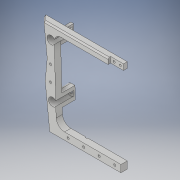
# Autodesk Inventor part: iPadGolf6Holder
Saved by Autodesk Inventor 2017 (Build 210142000, 142)
## iProperties
Created: 2022-11-09
Part Number: iPadGolf6Holder
Material: Generic
Document SubType Name: Modeling
Designer: khonsu
Density: 1 g/cm^3
Appearance: Default
Author: khonsu
Autodesk Inventor part; units mm, degrees
ref_plane "YZ Plane" through (0, 0, 0) normal (1, 0, 0) x (0, 1, 0)
ref_plane "XZ Plane" through (0, 0, 0) normal (0, 1, 0) x (-1, 0, 0)
sketch "Sketch1" plane through (0, 0, 0) normal (0, 0, 1) x (1, 0, 0)
  circle A0 centre (0, 0) radius 2.9
  line L0 (0, 0) -> (-2.42, 85.0556) construction
  line L1 (0, 0) -> (85.09, 0) construction
  line L2 (0, 0) -> (0, 165.0391) construction
  line L3 (-2.42, 85.0556) -> (0, 85.0556) construction
  circle A1 centre (-2.42, 85.0556) radius 2.9
  line L4 (0.48, 85.0556) -> (112.48, 85.0556) construction
  line L5 (112.48, 85.0556) -> (114.98, 85.0556) construction
  line L6 (-1.82, 94.7556) -> (2.68, 94.7556)
  line L7 (2.68, 85.6556) -> (2.68, 75.3556)
  line L8 (2.68, 75.3556) -> (-8.82, 75.3556)
  line L9 (-8.82, 75.3556) -> (-8.82, 87.7556)
  line L10 (-8.82, 87.6845) -> (1.18, 87.6845) construction
  line L11 (-1.4, -9.9) -> (5.7, -9.9)
  line L12 (5.7, -9.9) -> (5.7, 9.9)
  line L13 (5.7, 9.9) -> (-1.4, 9.9)
  line L14 (-6.4, 4.9) -> (-6.4, -4.9)
  arc A2 (-1.4, 9.9) -> (-6.4, 4.9) centre (-1.4, 4.9) ccw
  arc A3 (-6.4, -4.9) -> (-1.4, -9.9) centre (-1.4, -4.9) ccw
  line L15 (-1.82, 94.7556) -> (-8.82, 87.7556)
  line L16 (13.68, 96.6556) -> (114.98, 96.6556)
  line L17 (19.7, -32.2) -> (114.98, -32.2)
  line L18 (85.98, 105.8556) -> (114.98, 105.8556)
  line L19 (110.98, -43.7444) -> (114.98, -43.7444)
  line L20 (110.98, -43.7444) -> (-4.52, -43.7444)
  line L21 (110.98, -43.7444) -> (226.48, -43.7444) construction
  line L22 (85.98, 105.8556) -> (-20.72, 105.8556)
  line L23 (85.98, 105.8556) -> (192.68, 105.8556) construction
  line L24 (-20.72, 105.8556) -> (-4.52, -43.7444)
  line L25 (2.68, 96.6556) -> (2.68, 94.7556)
  line L26 (5.7, -18.2) -> (5.7, -9.9)
  arc A4 (13.68, 96.6556) -> (2.68, 85.6556) centre (13.68, 85.6556) ccw
  arc A5 (5.7, -18.2) -> (19.7, -32.2) centre (19.7, -18.2) ccw
  line L27 (114.98, 105.8556) -> (114.98, -43.7444)
  line L28 (2.68, 85.6556) -> (2.68, 94.7556)
  point P0 (-8.82, 94.7556)
  point P1 (5.7, -32.2)
  point P2 (-8.82, -58.1944)
  dimension "d5" = 5.8
  dimension "d0" = 5.8
  dimension "d1" = 85.09
  dimension "d3" = 2.42
  dimension "d4" = 0
  dimension "d6" = 112
  dimension "d7" = 2.5
  dimension "d10" = 9.7
  dimension "d11" = 6.4
  dimension "d12" = 5.1
  dimension "d13" = 9.7
  dimension "d16" = 0
  dimension "d18" = 6.4
  dimension "d19" = 9.9
  dimension "d20" = 9.9
  dimension "d21" = 5.7
  dimension "d22" = 5
  dimension "d23" = 7
  dimension "d24" = 7
  dimension "d25" = 1.9
  dimension "d26" = 0
  dimension "d27" = 0
  dimension "d28" = 22.3
  dimension "d29" = 0
  dimension "d30" = 0
  dimension "d31" = 149.6
  dimension "d32" = 9.2
  dimension "d33" = 4
  dimension "d34" = 0
  dimension "d35" = 115.5
  dimension "d36" = 180
  dimension "d37" = 29
  dimension "d38" = 0
  dimension "d39" = 106.7
  dimension "d40" = 180
  dimension "d41" = 11
  dimension "d42" = 14
  constraints: 58 end point, 13 horizontal, 9 tangent, 8 point on circle, 7 point on line, 5 centre point, 4 parallel, 4 perpendicular, 3 equal length, 2 coincident, 1 equal radius, 1 horizontal alignment, 1 vertical, 2 other
  measures "d0" diameter of A0
  measures "d1" distance of L0.start L0.end
  measures "d3" distance of L0.end L3.end
  measures "d4" distance from line of L2 L3.end
  measures "d6" distance of L4.start L4.end
  measures "d7" distance of L4.end L5.end
  measures "d10" distance from line of L6 point (-2.42, 85.056)
  measures "d11" distance from line of L9 point (-2.42, 85.056)
  measures "d12" distance from line of point (-2.42, 85.056) L7
  measures "d13" distance from line of L8 point (-2.42, 85.056)
  measures "d16" distance from line of L9 L10.start
  measures "d18" distance from line of L0.start L14
  measures "d19" distance from line of L11 L0.start
  measures "d20" distance from line of L13 L0.start
  measures "d21" distance from line of L12 L0.start
  measures "d22" radius of A2
  measures "d23" distance of L6.start point (-8.82, 94.756)
  measures "d24" distance of L9.end point (-8.82, 94.756)
  measures "d25" distance between parallel lines of L6 L16
  measures "d26" distance from line of L7 L25.start
  measures "d27" horizontal distance of L16.end L5.end
  measures "d28" distance between parallel lines of L11 L17
  measures "d29" distance from line of L12 point (5.7, -32.2)
  measures "d30" horizontal distance of L5.end L17.end
  measures "d31" distance between parallel lines of L19 L18
  measures "d32" distance between parallel lines of L16 L18
  measures "d33" distance of L19.start L19.end
  measures "d34" horizontal distance of L17.end L19.end
  measures "d35" distance of L19.start L20.end
  measures "d36" angle of L20 L21
  measures "d37" distance of L18.start L18.end
  measures "d38" horizontal distance of L16.end L18.end
  measures "d39" distance of L18.start L22.end
  measures "d40" angle of L22 L23
  measures "d41" radius of A4
  measures "d42" radius of A5
sketch "Sketch2" plane through (0, 0, 0) normal (1, 0, 0) x (0, 1, 0)
  line L0 (90.8641, 0) -> (90.8641, 21.12) construction
  line L1 (0, 0) -> (0, 31.12) construction
  dimension "d8" = 21.12
  dimension "d9" = 31.12
  constraints: 4 end point, 2 vertical
  measures "d8" distance of L0.start L0.end
  measures "d9" distance of L1.start L1.end
ref_plane "Work Plane2" through (0, 0, 31.12) normal (0, 0, 1) x (1, 0, 0)
sketch "Sketch4" plane through (0, 0, 31.12) normal (0, 0, 1) x (1, 0, 0)
  line L0 (3.18, 120.306) -> (114.98, 120.306)
  line L1 (114.98, 120.306) -> (114.98, -58.194)
  line L2 (114.98, -58.194) -> (3.18, -58.194)
  line L3 (-8.82, -46.194) -> (-8.82, 108.306)
  arc A0 (3.18, 120.306) -> (-8.82, 108.306) centre (3.18, 108.306) ccw
  arc A1 (-8.82, -46.194) -> (3.18, -58.194) centre (3.18, -46.194) ccw
  point P0 (0, 0)
  point P1 (-8.82, 120.306)
  dimension "d53" = 123.8
  dimension "d54" = 178.5
  dimension "d55" = 12
  dimension "d56" = 120.306
  dimension "d57" = 114.98
  constraints: 8 end point, 4 point on circle, 4 tangent, 2 centre point, 2 parallel, 2 point on line, 1 equal radius, 1 horizontal, 1 perpendicular
  measures "d53" distance of point (-8.82, 120.306) L0.end
  measures "d54" distance of L0.end L1.end
  measures "d55" radius of A0
  measures "d56" distance from line of point (0, 0) L0
  measures "d57" distance from line of L1 point (0, 0)
extrude "Extrusion1" add sketch "Sketch4" along normal blind 6.2
sketch "Sketch5" plane through (0, 0, 37.32) normal (0, 0, 1) x (1, 0, 0)
  line L0 (-30.2901, 140.4978) -> (261.1035, 140.4978) construction
  line L1 (261.1035, 140.4978) -> (261.1035, -78.1737) construction
  line L2 (261.1035, -78.1737) -> (-30.2901, -78.1737) construction
  line L3 (-30.2901, -78.1737) -> (-30.2901, 140.4978) construction
  line L4 (2.9472, 95.7116) -> (21.4756, 95.7116)
  line L5 (21.4756, 95.7116) -> (21.4756, 55.8918)
  line L6 (21.4756, 55.8918) -> (2.9472, 55.8918)
  line L7 (2.9472, 55.8918) -> (2.9472, 95.7116)
  line L8 (-5.1793, 84.9846) -> (1.4844, 84.9846)
  line L9 (1.4844, 84.9846) -> (1.4844, 67.7564)
  line L10 (1.4844, 67.7564) -> (-5.1793, 67.7564)
  line L11 (-5.1793, 67.7564) -> (-5.1793, 84.9846)
  line L12 (-5.1793, -10.2579) -> (1.4844, -10.2579)
  line L13 (1.4844, -10.2579) -> (1.4844, -27.486)
  line L14 (1.4844, -27.486) -> (-5.1793, -27.486)
  line L15 (-5.1793, -27.486) -> (-5.1793, -10.2579)
  line L16 (5.5477, 19.16) -> (22.6133, 19.16)
  line L17 (22.6133, 19.16) -> (22.6133, -33.4996)
  line L18 (22.6133, -33.4996) -> (5.5477, -33.4996)
  line L19 (5.5477, -33.4996) -> (5.5477, 19.16)
  line L20 (8.6767, 118.5205) -> (34.3813, 118.5205)
  line L21 (34.3813, 118.5205) -> (34.3813, 113.4913)
  line L22 (34.3813, 113.4913) -> (8.6767, 113.4913)
  line L23 (8.6767, 113.4913) -> (8.6767, 118.5205)
  line L24 (-1.8474, 113.4913) -> (21.4756, 113.4913)
  line L25 (21.4756, 113.4913) -> (21.4756, 89.4631)
  line L26 (21.4756, 89.4631) -> (-1.8474, 89.4631)
  line L27 (-1.8474, 89.4631) -> (-1.8474, 113.4913)
  arc A0 (3.4892, 119.7039) -> (-8.3493, 107.663) centre (3.3651, 107.9857) ccw
  line L28 (-8.82, 108.306) -> (-8.82, -46.194) projected
  line L29 (3.18, -58.194) -> (114.98, -58.194) projected
  arc A1 (-8.82, -46.194) -> (3.18, -58.194) centre (3.7792, -45.5948) ccw
  line L30 (-8.82, -46.194) -> (-8.82, 108.306)
  line L31 (114.98, 120.306) -> (3.18, 120.306) projected
  line L32 (3.18, 120.306) -> (85.0606, 120.306)
  line L33 (3.18, -58.194) -> (79.7167, -58.194)
  point P0 (0, 0)
  constraints: 54 end point, 13 equal length, 6 horizontal, 6 perpendicular, 6 point on line, 4 point on circle, 2 centre point, 2 other
extrude "Extrusion2" add sketch "Sketch1" along normal blind 2 contours L6 L28 L7 L8 L9 L15 | A3 L14 A2 L13 L12 L11
sketch "Sketch6" plane through (0, 0, 2) normal (0, 0, 1) x (1, 0, 0)
  circle A0 centre (-2.42, 85.0556) radius 2.9 projected
  circle A1 centre (-2.42, 85.0556) radius 6
  line L0 (-8.82, 87.7556) -> (-8.82, 75.3556) projected
  line L1 (-8.82, 75.3556) -> (2.68, 75.3556) projected
  line L2 (2.68, 81.5556) -> (2.68, 75.3556)
  line L3 (2.68, 75.3556) -> (-8.82, 75.3556)
  line L4 (-8.82, 75.3556) -> (-8.82, 81.5556)
  line L5 (2.68, 94.7556) -> (-1.82, 94.7556) projected
  line L6 (2.68, 94.7556) -> (-1.82, 94.7556)
  line L7 (-1.82, 94.7556) -> (-5.32, 91.2556)
  line L8 (-1.82, 94.7556) -> (-8.82, 87.7556) projected
  line L9 (-5.32, 91.2556) -> (2.68, 91.2556)
  line L10 (2.68, 75.3556) -> (2.68, 94.7556) projected
  line L11 (2.68, 94.7556) -> (2.68, 91.2556)
  circle A2 centre (0, 0) radius 2.9 projected
  arc A3 (5.7, 1.8735) -> (5.7, -1.8735) centre (0, 0) ccw
  arc A4 (-1.4, 9.9) -> (-6.4, 4.9) centre (-1.4, 4.9) ccw projected
  arc A5 (-1.4, 9.9) -> (-6.4, 4.9) centre (-1.4, 4.9) ccw
  arc A6 (-6.4, -4.9) -> (-1.4, -9.9) centre (-1.4, -4.9) ccw projected
  arc A7 (-6.4, -4.9) -> (-1.4, -9.9) centre (-1.4, -4.9) ccw
  line L12 (5.7, 9.9) -> (-1.4, 9.9) projected
  line L13 (5.7, 9.9) -> (-1.4, 9.9)
  line L14 (-6.4, 4.9) -> (-6.4, -4.9)
  line L15 (-1.4, -9.9) -> (5.7, -9.9)
  line L16 (5.7, -9.9) -> (5.7, 9.9)
  line L17 (-8.82, 81.5556) -> (-7.2934, 81.5556)
  line L18 (2.4534, 81.5556) -> (2.68, 81.5556)
  line L19 (-6.4, 4.9) -> (-6.4, -4.9) projected
  line L20 (-6.4, 4.9) -> (-6.4, -4.9)
  line L21 (-1.4, -9.9) -> (5.7, -9.9) projected
  line L22 (-1.4, -9.9) -> (5.7, -9.9)
  dimension "d103" = 12
  dimension "d104" = 12
  constraints: 30 end point, 12 point on circle, 6 parallel, 4 centre point, 4 perpendicular, 3 collinear, 3 horizontal, 3 point on line, 2 coincident, 2 concentric, 2 midpoint
  measures "d103" diameter of A1
  measures "d104" diameter of A3
extrude "Extrusion3" add sketch "Sketch6" along normal blind 19 contours A1 L18 L2 L1 L0 L17 | L9 L7 L5 L10 | A3 L16 L15 A6 L14 A4 L12
sketch "Sketch7" plane through (0, 0, 21) normal (0, 0, 1) x (1, 0, 0)
  line L0 (114.98, 105.8556) -> (-20.72, 105.8556)
  line L1 (-20.72, 105.8556) -> (-4.52, -43.7444)
  line L2 (-4.52, -43.7444) -> (114.98, -43.7444)
  line L3 (114.98, -43.7444) -> (114.98, -32.2001)
  line L4 (114.98, -32.2001) -> (19.3007, -32.2001)
  arc A0 (5.7019, -18.3639) -> (19.3007, -32.2001) centre (19.3007, -18.5993) ccw
  line L5 (5.7019, -18.3639) -> (2.68, 85.7253)
  line L6 (2.68, 81.5556) -> (2.68, 91.2556) projected
  arc A1 (13.6276, 96.6653) -> (2.68, 85.7253) centre (13.7375, 85.6078) ccw
  line L7 (13.6276, 96.6653) -> (114.98, 96.6653)
  line L8 (114.98, 96.6653) -> (114.98, 105.8556)
  circle A2 centre (-2.42, 85.0556) radius 2.9 projected
  arc A3 (2.9036, 87.8232) -> (2.786, 82.0728) centre (-2.42, 85.0556) ccw
  arc A4 (5.0759, 3.1993) -> (5.2529, -2.8994) centre (0, 0) ccw
  dimension "d107" = 135.7
  constraints: 16 end point, 9 point on circle, 4 centre point, 4 point on line, 3 perpendicular, 2 coincident, 2 horizontal, 1 parallel, 1 tangent
  measures "d107" distance of L0.start L0.end
extrude "Extrusion4" add sketch "Sketch7" along normal up to surface (10.12 mm away) contours L8 L7 A1 A3 L5 A4 A0 L4 L3 L2 L1 L0
sketch "Sketch13" plane through (-20.72, 105.8556, 31.12) normal (0, 0, 1) x (1, 0, 0)
  arc A0 (23.6236, -18.0324) -> (23.506, -23.7828) centre (18.3, -20.8) ccw projected
  circle A1 centre (18.3, -20.8) radius 6.5
  circle A2 centre (20.72, -105.8556) radius 6.5
  line L0 (26.4219, -124.2195) -> (25.9729, -108.755) projected
  line L1 (26.3194, -120.6899) -> (23.8978, -37.2782)
  line L2 (23.8978, -37.2782) -> (51.6668, -75.9953)
  line L3 (51.6668, -75.9953) -> (42.6037, -121.8387)
  line L4 (42.6037, -121.8387) -> (26.4219, -124.2195)
  dimension "d149" = 13
  dimension "d150" = 13
  constraints: 8 end point, 2 centre point, 2 coincident, 1 collinear, 1 point on line
  measures "d149" diameter of A1
  measures "d150" diameter of A2
extrude "Extrusion10" cut sketch "Sketch13" against normal up to surface (29.12 mm away) contours A1 | A2 L0 L1 | L1 L0 A2
extrude "Extrusion11" cut sketch "Sketch13" against normal blind 42.3875 contours A2 L0 L1 | A2 L1 L2 L3 L4 L0 picked at (26.1014, -104.5076)
sketch "Sketch20" plane through (0, 0, 37.32) normal (0, 0, 1) x (1, 0, 0)
  line L0 (-52.8355, 133.6203) -> (153.5294, 133.6203)
  line L1 (153.5294, 133.6203) -> (153.5294, -82.3162)
  line L2 (153.5294, -82.3162) -> (-52.8355, -82.3162)
  line L3 (-52.8355, -82.3162) -> (-52.8355, 133.6203)
  point P0 (0, 0)
  constraints: 8 end point, 2 parallel, 1 horizontal, 1 perpendicular
extrude "Extrusion20" cut sketch "Sketch20" against normal up to surface (6.2 mm away)
sketch "Sketch21" plane through (-20.72, 105.8556, 31.12) normal (0, 0, 1) x (1, 0, 0)
  circle A0 centre (120.7, -143.8278) radius 1.75
  circle A1 centre (95.7, -143.8278) radius 1.75
  circle A2 centre (70.7, -143.8278) radius 1.75
  circle A3 centre (17.5, -55) radius 1.75
  circle A4 centre (17.5, -80) radius 1.75
  line L0 (135.7, -138.0557) -> (135.7, -149.6) projected
  circle A5 centre (45.7, -143.8278) radius 1.75
  line L1 (0, 0) -> (135.7, 0) projected
  line L2 (130.7, 4.0811) -> (167.0922, 4.0811)
  line L3 (167.0922, 4.0811) -> (167.0922, -155.3274)
  line L4 (167.0922, -155.3274) -> (130.7, -155.3274)
  line L5 (130.7, -155.3274) -> (130.7, 4.0811)
  line L6 (135.7, 0) -> (135.7, -9.1902) projected
  circle A6 centre (125.7, -4.5951) radius 1.75
  circle A7 centre (115.7, -4.5951) radius 1.75
  point P0 (20.72, -105.8556)
  dimension "d194" = 3.5
  dimension "d195" = 3.5
  dimension "d196" = 3.5
  dimension "d197" = 3.5
  dimension "d198" = 3.5
  dimension "d199" = 15
  dimension "d200" = 25
  dimension "d201" = 25
  dimension "d202" = 3.5
  dimension "d203" = 25
  dimension "d204" = 55
  dimension "d205" = 25
  dimension "d206" = 5
  dimension "d207" = 3.5
  dimension "d208" = 3.5
  dimension "d209" = 10
  dimension "d210" = 10
  dimension "d213" = 17.5
  dimension "d214" = 0
  constraints: 8 centre point, 8 end point, 2 parallel, 1 horizontal, 1 perpendicular
  measures "d194" diameter of A0
  measures "d195" diameter of A1
  measures "d196" diameter of A2
  measures "d197" diameter of A3
  measures "d198" diameter of A4
  measures "d199" distance from line of L0 A0.centre
  measures "d200" distance of A0.centre A1.centre
  measures "d201" distance of A1.centre A2.centre
  measures "d202" diameter of A5
  measures "d203" distance of A2.centre A5.centre
  measures "d204" distance from line of L1 A3.centre
  measures "d205" distance of A3.centre A4.centre
  measures "d206" distance between parallel lines of L6 L5
  measures "d207" diameter of A6
  measures "d208" diameter of A7
  measures "d209" distance from line of L6 A6.centre
  measures "d210" distance of A6.centre A7.centre
  measures "d213" horizontal distance of L1.start A3.centre
  measures "d214" horizontal distance of A3.centre A4.centre
extrude "Extrusion21" cut sketch "Sketch21" against normal blind 16.35
chamfer "Chamfer6" distance 6.7625 angle 45 1 edges at (-12.62, 31.0556, 31.12)
sketch "Sketch23" plane through (19.3007, -32.2001, 31.12) normal (0, 0, 1) x (1, 0, 0)
  line L0 (-14.2508, 36.2925) -> (-16.4893, 113.398) projected
  line L1 (-17.0187, -11.5443) -> (90.6793, -11.5443) projected
  line L2 (-59.7546, 55.2057) -> (-59.7546, -11.5443)
  line L3 (-13.5988, 13.8362) -> (-14.0219, 28.4076) projected
  arc A0 (-14.2508, 36.2925) -> (-14.0219, 28.4076) centre (-19.3007, 32.2001) ccw
  arc A1 (-21.0787, 25.948) -> (-14.0219, 28.4076) centre (-19.3007, 32.2001) ccw projected
  line L4 (-14.7999, 55.2057) -> (-31.049, 55.2057)
  line L5 (-40.0207, 138.0557) -> (-23.8207, -11.5443) projected
  line L6 (90.6793, -11.5443) -> (-23.8207, -11.5443) projected
  line L7 (-31.049, 55.2057) -> (-23.8207, -11.5443)
  line L8 (-23.8207, -11.5443) -> (-12.862, -11.5443)
  line L9 (-14.7999, 55.2057) -> (-14.2508, 36.2925)
  line L10 (-14.0219, 28.4076) -> (-12.862, -11.5443)
  circle A2 centre (-22.5207, 83.0557) radius 1.75 projected
  circle A3 centre (-22.5207, 83.0557) radius 1.75
  line L11 (-28.2927, 88.8277) -> (-16.7487, 88.8277) construction
  line L12 (-16.7487, 88.8277) -> (-16.7487, 77.2837) construction
  line L13 (-16.7487, 77.2837) -> (-28.2927, 77.2837) construction
  line L14 (-28.2927, 77.2837) -> (-28.2927, 88.8277) construction
  circle A4 centre (-22.5207, 58.0557) radius 1.75 projected
  circle A5 centre (-22.5207, 58.0557) radius 1.75
  line L15 (-22.3759, 37.9267) -> (-33.2187, 138.0557) projected
  line L16 (-27.8879, 88.8277) -> (-31.049, 55.2057)
  line L17 (-31.049, 55.2057) -> (-14.7999, 55.2057)
  line L18 (-14.7999, 55.2057) -> (-16.7487, 88.8277)
  line L19 (-16.7487, 88.8277) -> (-27.8879, 88.8277)
  dimension "d231" = 0
  dimension "d232" = 66.75
  dimension "d233" = 0
  dimension "d234" = 0
  dimension "d244" = 5.772
  dimension "d245" = 5.772
  dimension "d246" = 5.772
  dimension "d247" = 5.772
  constraints: 28 end point, 3 centre point, 3 collinear, 3 horizontal, 3 point on circle, 3 point on line, 2 coincident, 2 parallel, 1 concentric, 1 perpendicular, 1 vertical
  measures "d231" distance from line of L1 L8.end
  measures "d232" distance of L2.start L2.end
  measures "d233" distance from line of L1 L2.end
  measures "d234" vertical distance of L4.start L2.start
  measures "d244" distance from line of A3.centre L11
  measures "d245" distance from line of L13 A3.centre
  measures "d246" distance from line of L12 A3.centre
  measures "d247" distance from line of L14 A3.centre
extrude "Extrusion23" add sketch "Sketch23" against normal up to surface (10.12 mm away) contours A0 L15 L4 L0 | A0 L3 L10 L1 L6 L5 L4 L15
chamfer "Chamfer8" distance 2.1825 angle 45 2 edges at (48.031, 105.8556, 31.12) (-17.319, 105.8556, 27.7388)
extrude "Extrusion24" add sketch "Sketch23" against normal up to surface (10.12 mm away) contours L4 L15 L19 L18 | L4 L16 L15
sketch "Sketch24" plane through (-4.52, -43.7444, 31.12) normal (0, -1, 0) x (1, 0, 0)
  arc A0 (50.9593, -10.62) -> (46.9593, -10.62) centre (48.9593, -10.62) ccw
  line L0 (114.5, -12.62) -> (0, -12.62) projected
  line L1 (0.7616, -12.62) -> (114.5, -12.62) projected
  line L2 (50.9593, -10.62) -> (50.9593, -12.62)
  line L3 (50.9593, -12.62) -> (46.9593, -12.62)
  line L4 (46.9593, -12.62) -> (46.9593, -10.62)
  point P0 (4.52, -31.12)
  dimension "d250" = 4
  dimension "d251" = 2
  constraints: 6 end point, 2 point on circle, 1 centre point, 1 parallel, 1 point on line
  measures "d250" diameter of A0
  measures "d251" distance from line of L0 A0.centre
extrude "Extrusion25" cut sketch "Sketch24" against normal blind 19.725
sketch "Sketch25" plane through (-6.4, -4.9, 0) normal (-1, 0, 0) x (0, 0, 1)
  line L0 (2, 7.8) -> (2, 2) projected
  line L1 (2, 7.8) -> (21, 7.8)
  line L2 (21, 7.8) -> (21, 2)
  line L3 (21, 2) -> (2, 2)
  line L4 (2, 2) -> (2, 7.8)
  line L5 (21, 3.7642) -> (21, 6.0358) projected
  point P0 (0, 4.9)
  dimension "d255" = 0
  dimension "d256" = 0
  constraints: 8 end point, 2 parallel, 1 horizontal, 1 perpendicular
  measures "d255" distance from line of L0.end L3
  measures "d256" distance between parallel lines of L5 L2
extrude "Extrusion26" cut sketch "Sketch25" against normal blind 10
sketch "Sketch26" plane through (-4.52, -43.7444, 31.12) normal (0, 0, 1) x (1, 0, 0)
  line L0 (93.728, 153.1062) -> (116.9342, 153.1062)
  line L1 (116.9342, 153.1062) -> (116.9342, 139.3839)
  line L2 (116.9342, 139.3839) -> (93.728, 139.3839)
  line L3 (93.728, 139.3839) -> (93.728, 153.1062)
  circle A0 centre (99.5, 145.0049) radius 1.75 projected
  circle A1 centre (99.5, 145.0049) radius 0.8453
  point P0 (4.52, 43.7444)
  dimension "d259" = 5.772
  constraints: 8 end point, 2 parallel, 1 centre point, 1 coincident, 1 horizontal, 1 perpendicular
  measures "d259" distance from line of A1.centre L3
extrude "Extrusion27" cut sketch "Sketch26" against normal blind 4 contours L0 L1 L2 L3 | A0 | A1
equation "\"d20\" = d19"
equation "\"d24\" = d23"
body "Solid1"
